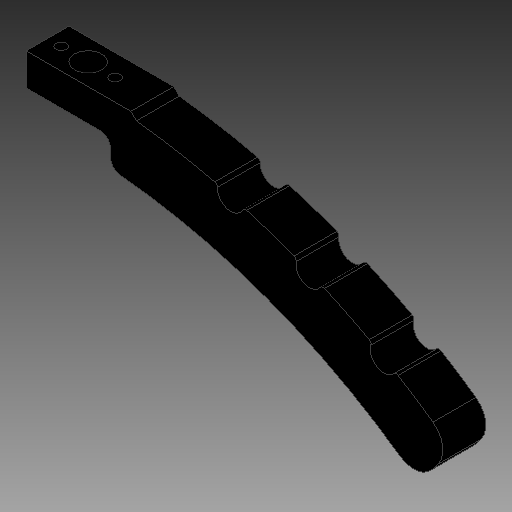
# Autodesk Inventor part: Arm Simplified
Saved by Autodesk Inventor 2019 (Build 230136000, 136)
## iProperties
Created: 2016-04-15
Part Number: Arm Simplified
Material: Aluminum 6061
Document SubType Name: Modeling
Designer: IEUser
Density: 2.7 g/cm^3
Appearance: Anodized - Black
Mass: 63.2332 g
Surface Area: 78.4771 cm^2
Volume: 23.4197 cm^3
Author: IEUser
Autodesk Inventor part; units mm, degrees
ref_plane "YZ Plane" through (0, 0, 0) normal (1, 0, 0) x (0, 1, 0)
ref_plane "XZ Plane" through (0, 0, 0) normal (0, 1, 0) x (-1, 0, 0)
ref_plane "XY Plane" through (0, 0, 0) normal (0, 0, 1) x (1, 0, 0)
sketch "Body Outline" plane through (0, 0, 0) normal (0, 0, 1) x (1, 0, 0)
  line L0 (0, 0) -> (31, 0)
  line L1 (31, 0) -> (32.6381, -1.6381)
  line L2 (0, 0) -> (0, -9.5)
  line L3 (0, -9.5) -> (25, -9.5)
  line L4 (25, -9.5) -> (25, -17.6949)
  arc A0 (126.2645, -39.2876) -> (32.6381, -1.6381) centre (12, -188.2) ccw
  arc A1 (116.0982, -52.5366) -> (25, -17.6949) centre (12, -188.2) ccw
  line L5 (116.0982, -52.5366) -> (126.2645, -39.2876)
  dimension "d0" = 45
  dimension "d1" = 0
  dimension "d2" = 0
  dimension "d3" = 9.5
  dimension "d4" = 171
  dimension "d5" = 187.7
  dimension "d6" = 37.5
  dimension "d7" = 12
  dimension "d8" = 188.2
  dimension "d9" = 25
  dimension "d10" = 31
  constraints: 12 end point, 4 point on circle, 2 centre point, 2 perpendicular, 1 concentric, 1 horizontal, 1 line through centre, 1 vertical
  measures "d0" angle of L1 L0
  measures "d1" distance from line of point (0, 0) L2
  measures "d2" distance from line of point (0, 0) L0
  measures "d3" distance of L0.start L2.end
  measures "d4" radius of A1
  measures "d5" radius of A0
  measures "d6" angle of L5 L4
  measures "d7" distance from line of L2 A0.centre
  measures "d8" distance from line of L0 A0.centre
  measures "d9" distance between parallel lines of L4 L2
  measures "d10" distance of L0.start L0.end
extrude "Body" add sketch "Body Outline" along normal mid plane 12.7
sketch "Dowel Pin Hole Positions" plane through (0, 0, 6.35) normal (0, 1, 0) x (1, 0, 0)
  line L0 (0, 12.7) -> (0, 0) projected
  point P0 (0, 6.35)
  point P1 (4, 6.35)
  point P2 (20, 6.35)
  dimension "d13" = 0
  dimension "d14" = 4
  dimension "d15" = 0
  dimension "d16" = 20
  measures "d13" vertical distance of point (0, 6.35) point (4, 6.35)
  measures "d14" distance from line of L0 point (4, 6.35)
  measures "d15" vertical distance of point (0, 6.35) point (20, 6.35)
  measures "d16" distance from line of L0 point (20, 6.35)
hole "Dowel Pin Holes" at (4, 0, 0) at (20, 0, 0) direction (0, -1, 0) diameter 2 end through all counterbore diameter 3.1 counterbore depth 7
sketch "Fastening Hole Position" plane through (0, 0, 6.35) normal (0, 1, 0) x (1, 0, 0)
  line L0 (0, 12.7) -> (0, 0) projected
  point P0 (0, 6.35)
  point P1 (12, 6.35)
  dimension "d24" = 0
  dimension "d25" = 12
  measures "d24" vertical distance of point (0, 6.35) point (12, 6.35)
  measures "d25" distance from line of point (12, 6.35) L0
hole "Fastening Hole" at (12, 0, 0) direction (0, -1, 0) diameter 8.1 end through all
sketch "Thumbscrew Cutout Outline" plane through (0, 0, 6.35) normal (0, 0, 1) x (1, 0, 0)
  arc A0 (126.2645, -39.2876) -> (32.6381, -1.6381) centre (12, -188.2) ccw projected
  line L0 (54.964, -27.8563) -> (60.5803, -6.8957) construction
  line L1 (0, 0) -> (0, -9.5) projected
  arc A1 (60.5803, -6.8957) -> (28.3591, -1.2143) centre (12, -188.2) ccw construction
  line L2 (12, -188.2) -> (28.3591, -1.2143) construction
  line L3 (12, -188.2) -> (60.5803, -6.8957) construction
  arc A2 (54.964, -27.8563) -> (26.4679, -22.8317) centre (12, -188.2) ccw construction
  line L4 (12, -188.2) -> (26.4679, -22.8317) construction
  line L5 (12, -188.2) -> (54.964, -27.8563) construction
  circle A3 centre (60.5803, -6.8957) radius 4
  dimension "d50" = 15
  dimension "d51" = 10
  dimension "d52" = 10
  dimension "d53" = 166
  dimension "d54" = 187.7
  dimension "d67" = 8
  constraints: 10 end point, 4 point on circle, 3 centre point, 2 concentric, 1 coincident, 1 line through centre
  measures "d50" angle of L1 L0
  measures "d51" angle of L3 L2
  measures "d52" angle of L5 L4
  measures "d53" radius of A2
  measures "d54" radius of A1
  measures "d67" diameter of A3
extrude "Thumbscrew Cutout" cut sketch "Thumbscrew Cutout Outline" against normal through all
pattern_circular "Thumbscrew Cutout Pattern" count 3 over 15 about axis through (12, -188.2, 0) along (0, 0, -1) of "Thumbscrew Cutout"
fillet "Body Fillet" radius 1 6 edges at (56.7058, -5.9017, 0) (64.4328, -7.9721, 0) (80.1181, -13.2965, 0) (87.5087, -16.3578, 0) (102.3648, -23.6841, 0) (109.2926, -27.6838, 0)
fillet "Body Fillet" radius 3 2 edges at (25, -9.5, 0) (25, -17.6949, 0)
fillet "Body Fillet" radius 7 2 edges at (126.2645, -39.2876, 0) (116.0982, -52.5366, 0)
equation "\"d54\" = d5"
body "Solid1"
